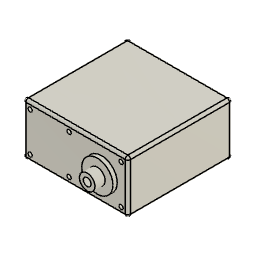
STS3020双轴舵机 v1 (Autodesk Fusion 360 design; units mm, degrees)
Autodesk Fusion 360 part; units mm, degrees
note: some values were not read from the file. Set by a fixed rule: which sketch regions a step uses.
sketch "草图1" plane through (0, 0, 0) normal (0, 1, 0) x (1, 0, 0)
  line L0 (0, 0) -> (40.2, 0)
  line L1 (40.2, 0) -> (40.2, -20.2)
  line L2 (40.2, -20.2) -> (0, -20.2)
  line L3 (0, -20.2) -> (0, 0)
  dimension "d1" = 20.2
  dimension "d2" = 40.2
  constraint horizontal L0
  constraint vertical L1
  constraint horizontal L2
  constraint vertical L3
  constraint coincident L0.start L3.end
  measures "d1" distance of L0.end L1.end
  measures "d2" distance of L0.start L0.end
extrude "拉伸1" add sketch "草图1" along normal blind 40.1 makes body 1
sketch "草图2" plane through (0, 0, 0) normal (0, -1, 0) x (1, 0, 0)
  line L0 (40.2, 20.2) -> (0, 20.2)
  line L1 (0, 20.2) -> (0, 0)
  line L2 (0, 0) -> (40.2, 0)
  line L3 (40.2, 0) -> (40.2, 20.2)
  line L4 (20.1, 23) -> (20.1, -21)
  line L5 (2.071, 10.1) -> (35, 10.1)
  circle A0 centre (2.6, 17.6) radius 0.8
  circle A1 centre (37.6, 17.6) radius 0.8
  circle A2 centre (2.6, 2.6) radius 0.8
  circle A3 centre (37.6, 2.6) radius 0.8
  circle A4 centre (17.6, 17.6) radius 0.8
  circle A5 centre (17.6, 2.6) radius 0.8
  dimension "d5" = 1.6
  dimension "d6" = 15
  dimension "d7" = 35
  dimension "d8" = 1.6
  dimension "d9" = 5
  dimension "d12" = 15
  constraint perpendicular L0 L4
  constraint symmetric L1 L3 L4
  constraint perpendicular L4 L5
  constraint symmetric L4 A0 A1
  constraint symmetric L5 A0 A2
  constraint symmetric L5 A1 A3
  constraint symmetric L5 A4 A5
  measures "d5" diameter of A0
  measures "d6" distance of A0.centre A2.centre
  measures "d8" diameter of A4
  measures "d12" distance of A4.centre A5.centre
extrude "拉伸2" cut sketch "草图2" against normal blind 4 contours A0 | A1 | A2 | A3 | A4 | A5 bodies 1
sketch "草图3" plane through (0, 0, 0) normal (0, -1, 0) x (1, 0, 0)
  circle A0 centre (17.6, 2.6) radius 0.8
  circle A1 centre (2.6, 17.6) radius 0.8
  circle A2 centre (37.6, 17.6) radius 0.8
  circle A3 centre (17.6, 17.6) radius 0.8
  circle A4 centre (2.6, 2.6) radius 0.8
  circle A5 centre (37.6, 2.6) radius 0.8
  line L0 (40.2, 20.2) -> (0, 20.2)
  line L1 (0, 20.2) -> (0, 0)
  line L2 (0, 0) -> (40.2, 0)
  line L3 (40.2, 0) -> (40.2, 20.2)
  line L4 (20.1, 18.9238) -> (20.1, 1)
  circle A6 centre (30.1, 9.9619) radius 6
  dimension "d13" = 12
  dimension "d29" = 20
  constraint perpendicular L0 L4
  constraint symmetric L1 L3 L4
  measures "d13" diameter of A6
extrude "拉伸3" add sketch "草图3" along normal blind 1.65 contours A6 bodies 1
sketch "草图4" plane through (0, -1.65, 0) normal (0, -1, 0) x (1, 0, 0)
  circle A0 centre (30.1, 9.9619) radius 6
  circle A1 centre (30.1, 9.9619) radius 3
  dimension "d16" = 6
  constraint concentric A0 A1
  measures "d16" diameter of A1
extrude "拉伸4" add sketch "草图4" along normal blind 3.9 contours A1 bodies 1
sketch "草图5" plane through (0, 40.1, 0) normal (0, 1, 0) x (-1, 0, 0)
  line L0 (0, 20.2) -> (-40.2, 20.2)
  line L1 (-40.2, 20.2) -> (-40.2, 0)
  line L2 (-40.2, 0) -> (0, 0)
  line L3 (0, 0) -> (0, 20.2)
  line L4 (-20.1, 1) -> (-20.1, 25)
  circle A0 centre (-30.1, 10) radius 6
  dimension "d19" = 12
  dimension "d20" = 20
  constraint vertical L4
  constraint symmetric L1 L3 L4
  measures "d19" diameter of A0
extrude "拉伸5" add sketch "草图5" along normal blind 1.65 contours A0 bodies 1
sketch "草图6" plane through (0, 41.75, 0) normal (0, 1, 0) x (-1, 0, 0)
  circle A0 centre (-30.1, 10) radius 6
  circle A1 centre (-30.1, 10) radius 3
  dimension "d23" = 6
  constraint concentric A0 A1
  measures "d23" diameter of A1
extrude "拉伸6" add sketch "草图6" along normal blind 4.1 contours A1 bodies 1
sketch "草图7" plane through (0, 45.85, 0) normal (0, 1, 0) x (-1, 0, 0)
  circle A0 centre (-30.1, 10) radius 3
  circle A1 centre (-30.1, 10) radius 1.5
  dimension "d26" = 3
  constraint concentric A0 A1
  measures "d26" diameter of A1
extrude "拉伸7" cut sketch "草图7" against normal blind 6 contours A1 bodies 1
sketch "草图8" plane through (0, 40.1, 0) normal (0, 1, 0) x (-1, 0, 0)
  circle A0 centre (-30.1, 10) radius 6
  line L0 (0, 20.2) -> (-40.2, 20.2)
  line L1 (-40.2, 20.2) -> (-40.2, 0)
  line L2 (-40.2, 0) -> (0, 0)
  line L3 (0, 0) -> (0, 20.2)
  line L4 (-20.1, 25.0001) -> (-20.1, -10.3333)
  circle A1 centre (-2.95, 10) radius 0.8
  line L5 (-39, 10) -> (5, 10)
  circle A2 centre (-9.95, 15.167) radius 0.8
  circle A3 centre (-9.95, 4.833) radius 0.8
  dimension "d30" = 1.6
  dimension "d31" = 34.3
  dimension "d32" = 1.6
  dimension "d33" = 7
  constraint symmetric L1 L3 L4
  constraint horizontal L5
  constraint symmetric L5 A2 A3
  measures "d30" diameter of A1
  measures "d32" diameter of A2
  measures "d33" horizontal distance of A1.centre A2.centre
extrude "拉伸8" cut sketch "草图8" against normal blind 6 contours A1 L5 | A1 L5 | A2 | A3 bodies 1
fillet "圆角1" radius 1 12 edges at (40.2, 20.05, 20.2) (40.2, 40.1, 10.1) (40.2, 20.05, 0) (40.2, 0, 10.1) (20.1, 40.1, 0) (20.1, 40.1, 20.2) (20.1, 0, 20.2) (20.1, 0, 0) (0, 20.05, 20.2) (0, 40.1, 10.1) (0, 20.05, 0) (0, 0, 10.1) on bodies 1
sketch "草图9" plane through (0, -5.55, 0) normal (0, -1, 0) x (1, 0, 0)
  circle A0 centre (30.1, 9.9619) radius 3
  circle A1 centre (30.1, 9.9619) radius 1.5
  dimension "d38" = 3
  constraint concentric A0 A1
  measures "d38" diameter of A1
extrude "拉伸9" cut sketch "草图9" against normal blind 6 contours A1 bodies 1
copy_body "实体->零部件1" bodies 1 removing the originals makes body 2 in component "Component'"
component "Component'" placed x (1, 0, 0) y (0, 1, 0) z (0, 0, 1) at (0, 0, 0)
